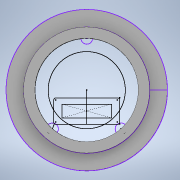
# Autodesk Inventor part: fingerprint sensor seal
Saved by Autodesk Inventor 2022 (Build 260153000, 153)
## iProperties
Created: 2022-06-08
Part Number: fingerprint sensor seal
Material: Generic
Document SubType Name: Modeling
Designer: alecw
Density: 1 g/cm^3
Appearance: Default
Author: alecw
Autodesk Inventor part; units mm, degrees
ref_plane "YZ Plane" through (0, 0, 0) normal (1, 0, 0) x (0, 1, 0)
ref_plane "XZ Plane" through (0, 0, 0) normal (0, 1, 0) x (-1, 0, 0)
ref_plane "XY Plane" through (0, 0, 0) normal (0, 0, 1) x (1, 0, 0)
sketch "Sketch1" plane through (0, 0, 0) normal (0, 0, 1) x (1, 0, 0)
  circle A0 centre (0, 0) radius 9.4
  circle A1 centre (0, 0) radius 10.45
  circle A2 centre (0, 0) radius 7
  line L0 (0, 0) -> (0, 1.4)
  line L1 (0, 1.4) -> (-5.6, 1.4)
  line L2 (-6, 1.8) -> (-6, 5.8)
  line L3 (-5.6, 6.2) -> (0, 6.2)
  arc A3 (-6, 1.8) -> (-5.6, 1.4) centre (-5.6, 1.8) ccw
  arc A4 (-5.6, 6.2) -> (-6, 5.8) centre (-5.6, 5.8) ccw
  line L4 (0, 1.4) -> (5.6, 1.4)
  line L5 (6, 1.8) -> (6, 5.8)
  line L6 (5.6, 6.2) -> (0, 6.2)
  arc A5 (5.6, 1.4) -> (6, 1.8) centre (5.6, 1.8) ccw
  arc A6 (6, 5.8) -> (5.6, 6.2) centre (5.6, 5.8) ccw
  circle A7 centre (0, -9.4) radius 1.05
  line L7 (5.8828, 6.0828) -> (6.2306, 7.0384)
  line L8 (5.8828, 6.0828) -> (6.8997, 6.0828) construction
  circle A8 centre (6.2306, 7.0384) radius 1.0741
  circle A9 centre (-6.2306, 7.0384) radius 1.0741
  line L9 (0, 6.2) -> (0, 1.4)
  line L10 (-4.5, 2.55) -> (4.5, 2.55)
  line L11 (4.5, 2.55) -> (4.5, 5.05)
  line L12 (4.5, 5.05) -> (-4.5, 5.05)
  line L13 (-4.5, 5.05) -> (-4.5, 2.55)
  line L14 (-4.5, 2.55) -> (4.5, 5.05) construction
  line L15 (4.5, 2.55) -> (-4.5, 5.05) construction
  line L16 (-10.45, 0) -> (-11.45, 0)
  circle A10 centre (0, 0) radius 11.45
  line L17 (-11.45, 0) -> (-14.65, 0)
  circle A11 centre (0, 0) radius 14.65
  point P0 (-6, 1.4)
  point P1 (-6, 6.2)
  point P2 (1.0484, -9.3414)
  point P3 (-1.0484, -9.3414)
  point P4 (7.1035, 7.6644)
  point P5 (6.7461, 7.9808)
  point P6 (5.387, 7.7033)
  point P7 (6.9929, 6.2816)
  point P8 (-7.1035, 7.6644)
  point P9 (-6.9929, 6.2816)
  point P10 (-5.387, 7.7033)
  point P11 (-6.7461, 7.9808)
  point P12 (0, 3.8)
  dimension "d1" = 20.9
  dimension "d0" = 18.8
  dimension "d8" = 14
  dimension "d18" = 1.4
  dimension "d19" = 6
  dimension "d20" = 4.8
  dimension "d21" = 0.4
  dimension "d22" = 70
  dimension "d25" = 9
  dimension "d26" = 2.5
  dimension "d31" = 1
  dimension "d32" = 3.2
  constraints: 36 end point, 11 point on circle, 9 centre point, 7 symmetric about line, 6 coincident, 4 horizontal, 4 point on line, 4 tangent, 3 midpoint, 3 perpendicular, 3 vertical, 2 horizontal alignment, 2 parallel, 1 equal length, 1 equal radius, 10 other
  measures "d0" diameter of A0
  measures "d8" diameter of A2
  measures "d18" distance of L0.start L0.end
  measures "d19" distance of L0.end point (-6, 1.4)
  measures "d20" distance of point (-6, 1.4) point (-6, 6.2)
  measures "d21" radius of A3
  measures "d22" angle of L8 L7
  measures "d25" distance of L12.end L11.end
  measures "d26" distance of L11.end L10.end
  measures "d31" distance of L16.start L16.end
  measures "d32" distance of L16.end L17.end
extrude "Extrusion7" add sketch "Sketch1" along normal blind 1.7 contours A0 A8 A1 A7 | A0 A8 A1 | A7 A0 | A7 A1 A9 A0 | A0 A9 A1 A8 | A9 A1 A0 | A10 picked at (0, -9.7457)
extrude "Extrusion8" add sketch "Sketch1" against normal blind 3.2 from surface at 0 contours A10
extrude "Extrusion9" add sketch "Sketch1" against normal blind 1 from surface at -3.2 contours A10 | A11
body "Solid2"
